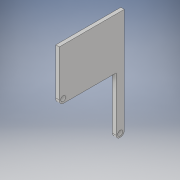
# Autodesk Inventor part: Ventilador bobina - suport
Saved by Autodesk Inventor 2019 (Build 230136000, 136)
## iProperties
Created: 2018-09-18
Part Number: Ventilador bobina - suport
Material: Genérico
Document SubType Name: Modeling
Designer: Albert Garangou Culebras
Density: 1 g/cm^3
Appearance: Valor por defecto
Author: Albert Garangou Culebras
Autodesk Inventor part; units mm, degrees
ref_plane "YZ Plane" through (0, 0, 0) normal (1, 0, 0) x (0, 1, 0)
ref_plane "XZ Plane" through (0, 0, 0) normal (0, 1, 0) x (-1, 0, 0)
ref_plane "XY Plane" through (0, 0, 0) normal (0, 0, 1) x (1, 0, 0)
sketch "Boceto1" plane through (0, 0, 0) normal (1, 0, 0) x (0, 1, 0)
  line L0 (3, 2.8622) -> (44, 2.8622)
  line L1 (50, 0) -> (50, -3)
  line L2 (3, -3) -> (3, 2.8622)
  line L3 (3, -3) -> (50, -3)
  circle A0 centre (5.75, -0.0689) radius 1.75
  line L4 (50, 43) -> (44, 43)
  line L5 (44, 43) -> (44, 2.8622)
  line L6 (50, 43) -> (50, 0)
  circle A1 centre (47, 40.25) radius 1.75
  point P0 (0, 0)
  constraints: 16 end point, 2 centre point, 2 perpendicular, 2 vertical, 1 horizontal
sketch "Boceto2" plane through (0, 0, 0) normal (1, 0, 0) x (0, 1, 0)
  line L0 (65, -3) -> (50, -3)
  line L1 (65, 43) -> (50, 43)
  line L2 (50, 43) -> (50, -3)
  line L3 (65, 43) -> (65, -3)
  point P0 (0, 0)
  constraints: 8 end point, 1 vertical
extrude "Extrusión3" [suppressed]
extrude "Extrusión5" add sketch "Boceto1" along normal blind 2.5
fillet "Empalme5" radius 3.5 1 edges at (1.25, 44, 43) curvature continuous yes
fillet "Empalme6" radius 2.9 2 edges at (1.25, 3, -3) (1.25, 3, 2.8622)
extrude "Extrusión6" add sketch "Boceto2" along normal blind 2.5
sketch "Boceto3" plane through (2.5, 0, 0) normal (1, 0, 0) x (0, 0, -1)
  line L0 (-43, 65) -> (-43, 47.5) projected
  line L1 (-43, 65) -> (-43, 70)
  line L2 (-43, 70) -> (3, 70)
  line L3 (3, 5.9) -> (3, 65) projected
  line L4 (3, 70) -> (3, 65)
  line L5 (3, 65) -> (-43, 65) projected
  line L6 (3, 65) -> (-43, 65)
  point P0 (0, 0)
  dimension "d36" = 5
  constraints: 8 end point, 2 perpendicular, 1 collinear, 1 vertical
  measures "d36" distance of L0.start L1.end
extrude "Extrusión7" add sketch "Boceto3" against normal blind 2.5
sketch "Boceto4" plane through (2.5, 70, 43) normal (0, 1, 0) x (1, 0, 0)
  line L0 (-2.5, 0) -> (-2.5, 46) projected
  line L1 (-2.5, 0) -> (0, 0)
  line L2 (0, 0) -> (0, 46)
  line L3 (0, 46) -> (-2.5, 46)
  line L4 (-2.5, 46) -> (-2.5, 0)
  point P0 (-2.5, 43)
  constraints: 8 end point, 2 parallel, 1 horizontal, 1 perpendicular
extrude "Extrusión8" add sketch "Boceto4" along normal blind 10
